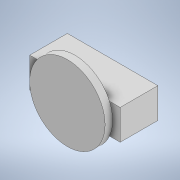
# Autodesk Inventor part: MinusBtn
Saved by Autodesk Inventor 2020.1 (Build 241239000, 239)
## iProperties
Created: 2019-09-04
Part Number: MinusBtn
Material: Generic
Document SubType Name: Modeling
Designer: matteo.spadetto-1
Density: 1 g/cm^3
Appearance: Default
Author: matteo.spadetto-1
Autodesk Inventor part; units mm, degrees
ref_plane "YZ Plane" through (0, 0, 0) normal (1, 0, 0) x (0, 1, 0)
ref_plane "XZ Plane" through (0, 0, 0) normal (0, 1, 0) x (-1, 0, 0)
ref_plane "XY Plane" through (0, 0, 0) normal (0, 0, 1) x (1, 0, 0)
sketch "Sketch1" plane through (0, 0, 0) normal (0, 0, 1) x (1, 0, 0)
  line L0 (0, 6) -> (0, 8)
  line L1 (0, 8) -> (12, 8)
  line L2 (12, 8) -> (12, 4)
  line L3 (12, 4) -> (0, 4)
  line L4 (0, 6) -> (0, 4)
  point P0 (0, 0)
  dimension "d2" = 2
  dimension "d3" = 4
  constraints: 10 end point, 1 vertical
  measures "d2" distance of L0.start L0.end
  measures "d3" distance of L1.end L2.end
extrude "Extrusion1" add sketch "Sketch1" along normal blind 5
sketch "Sketch2" plane through (0, 0, 5) normal (0, 0, 1) x (1, 0, 0)
  line L0 (0, 8) -> (0, 4) projected
  line L1 (12, 4) -> (12, 8) projected
  line L2 (12, 8) -> (0, 8) projected
  line L3 (0, 4) -> (12, 4) projected
  line L4 (0, 6) -> (12, 6)
  line L5 (6, 8) -> (6, 4)
  circle A0 centre (6, 6) radius 5
  point P0 (0, 0)
  dimension "d9" = 10
  constraints: 5 midpoint, 4 end point, 1 centre point
  measures "d9" diameter of A0
extrude "Extrusion3" add sketch "Sketch2" along normal blind 1 contours A0 L2 | L2 L5 L4 A0 | L4 L5 L3 A0 | L2 A0 L4 L5 | L3 A0 | L4 A0 L3 L5
body "Solid1"
